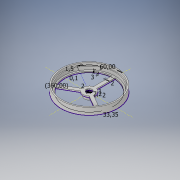
# Autodesk Inventor part: ShaftHolder
Saved by Autodesk Inventor 2018.3 (Build 223284000, 284)
## iProperties
Created: 2018-07-23
Part Number: ShaftHolder
Material: Generisch
Document SubType Name: Modeling
Designer: JochenAlt
Density: 1 g/cm^3
Appearance: Vorgabe
Author: JochenAlt
Autodesk Inventor part; units mm, degrees
ref_plane "YZ Plane" through (0, 0, 0) normal (1, 0, 0) x (0, 1, 0)
ref_plane "XZ Plane" through (0, 0, 0) normal (0, 1, 0) x (-1, 0, 0)
ref_plane "XY Plane" through (0, 0, 0) normal (0, 0, 1) x (1, 0, 0)
sketch "Skizze1" plane through (0, 0, 0) normal (0, 0, 1) x (1, 0, 0)
  circle A0 centre (0, 0) radius 33.35 construction
  circle A1 centre (0, 0) radius 34.95
  circle A2 centre (0, 0) radius 3.6
  circle A3 centre (0, 0) radius 5.6
  circle A4 centre (0, 0) radius 33.45
  circle A5 centre (0, 0) radius 2.6
  line L0 (0, 51.4164) -> (0, -49.3444) construction
  line L1 (-54.4561, 0) -> (54.4561, 0) construction
  line L2 (-2, 30.284) -> (-2, 7.3321)
  line L3 (0, 0) -> (-28.9685, 16.725) construction
  line L4 (-27.2267, -13.41) -> (-7.3498, -1.934)
  arc A6 (-2, 7.3321) -> (-7.3498, -1.934) centre (0, 0) ccw
  arc A7 (-2, 30.284) -> (-27.2267, -13.41) centre (0, 0) ccw
  line L5 (25.2267, -16.8741) -> (5.3498, -5.3981)
  arc A8 (-25.2267, -16.8741) -> (25.2267, -16.8741) centre (0, 0) ccw
  line L6 (-25.2267, -16.8741) -> (-5.3498, -5.3981)
  arc A9 (-5.3498, -5.3981) -> (5.3498, -5.3981) centre (0, 0) ccw
  line L7 (2, 30.284) -> (2, 7.3321)
  arc A10 (27.2267, -13.41) -> (2, 30.284) centre (0, 0) ccw
  line L8 (27.2267, -13.41) -> (7.3498, -1.934)
  arc A11 (7.3498, -1.934) -> (2, 7.3321) centre (0, 0) ccw
  circle A12 centre (0, 0) radius 32.35
  dimension "d1" = 33.35
  dimension "d2" = 7.2
  dimension "d3" = 2
  dimension "d4" = 0.1
  dimension "d5" = 1.5
  dimension "d12" = 1
  dimension "d17" = 60
  dimension "d18" = 2
  dimension "d19" = 3
  dimension "d20" = 2
  dimension "d23" = 360
  dimension "d25" = 1
  constraints: 14 end point, 12 centre point, 12 point on circle, 9 coincident, 1 vertical, 35 other
  measures "d1" radius of A0
  measures "d2" diameter of A2
  measures "d3" radial gap between concentric circles of A3 A2
  measures "d12" radial gap between concentric circles of A2 A5
  measures "d17" angle of L0 L3
  measures "d18" radial gap between concentric circles of A6 A3
  measures "d19" radial gap between concentric circles of A7 A0
  measures "d20" distance between parallel lines of L0 L2
  measures "d25" radial gap between concentric circles of A0 A12
extrude "Extrusion1" add sketch "Skizze1" along normal blind 1.5 contours A1 | A3 | A4 | A12
extrude "Extrusion2" add sketch "Skizze1" along normal blind 7 from surface at 1.5 contours A1
extrude "Extrusion3" add sketch "Skizze1" against normal blind 3 from surface at 0 contours A3
extrude "Extrusion4" add sketch "Skizze1" against normal blind 1.5 from surface at -3 contours A2 | A3
extrude "Extrusion5" add sketch "Skizze1" along normal blind 4 from surface at 1.5 contours A4
